Autodesk Fusion 360 part; units mm, degrees
(part 4 of 7)
  spline S889 degree 3 poles (-27.7984, 38.7746) (-27.7984, 38.6069) (-27.5964, 38.6069) (-27.5964, 38.7412) knots 0 0 0 0 1 1 1 1
  spline S890 degree 3 poles (-27.5964, 38.7412) (-27.5964, 38.8756) (-27.4117, 39.3291) (-27.4117, 38.7918) knots 0 0 0 0 1 1 1 1
  spline S891 degree 3 poles (-27.4117, 38.7918) (-27.4117, 38.6069) (-27.2945, 38.7079) (-27.2945, 38.809) knots 0 0 0 0 1 1 1 1
  line L641 (-27.2945, 38.809) -> (-27.2903, 38.9208)
  spline S892 degree 3 poles (-27.2903, 38.9208) (-27.2569, 39.1227) (-27.3826, 39.1603) (-27.4986, 39.2635) knots 0 0 0 0 1 1 1 1
  spline S893 degree 3 poles (-25.8872, 39.0304) (-25.9226, 39.5849) (-26.1773, 40.0898) (-26.6436, 40.5347) knots 0 0 0 0 1 1 1 1
  spline S894 degree 2 poles (-26.6436, 40.5347) (-26.578, 40.3295) (-26.5694, 40.0962) knots 0 0 0 1 1 1
  spline S895 degree 2 poles (-26.5694, 40.0962) (-26.6361, 40.2618) (-26.8208, 40.1779) knots 0 0 0 1 1 1
  spline S896 degree 2 poles (-26.8208, 40.1779) (-26.7198, 39.9598) (-26.7541, 39.7245) knots 0 0 0 1 1 1
  spline S897 degree 2 poles (-26.7541, 39.7245) (-26.8208, 39.8589) (-26.9218, 39.8922) knots 0 0 0 1 1 1
  spline S898 degree 2 poles (-26.9218, 39.8922) (-26.838, 39.7407) (-26.8551, 39.5063) knots 0 0 0 1 1 1
  spline S899 degree 2 poles (-26.8551, 39.5063) (-26.939, 39.6406) (-27.0905, 39.5902) knots 0 0 0 1 1 1
  spline S900 degree 2 poles (-27.0905, 39.5902) (-27.0572, 39.4731) (-27.0733, 39.271) knots 0 0 0 1 1 1
  spline S901 degree 2 poles (-27.0733, 39.271) (-27.157, 39.4407) (-27.2913, 39.3377) knots 0 0 0 1 1 1
  spline S902 degree 2 poles (-27.2913, 39.3377) (-27.0733, 39.0861) (-27.1065, 38.5651) knots 0 0 0 1 1 1
  spline S903 degree 3 poles (-27.1065, 38.5651) (-27.0077, 38.6527) (-26.9424, 38.7719) (-26.9218, 38.9025) knots 0 0 0 0 1 1 1 1
  spline S904 degree 2 poles (-26.9218, 38.9025) (-26.8884, 38.8165) (-26.8208, 38.6993) knots 0 0 0 1 1 1
  spline S905 degree 2 poles (-26.8208, 38.6993) (-26.7875, 38.768) (-26.7369, 38.9507) knots 0 0 0 1 1 1
  spline S906 degree 2 poles (-26.7369, 38.9507) (-26.6532, 38.6672) (-26.6704, 38.464) knots 0 0 0 1 1 1
  spline S907 degree 2 poles (-26.6704, 38.464) (-26.519, 38.7832) (-26.5694, 39.2366) knots 0 0 0 1 1 1
  spline S908 degree 2 poles (-26.5694, 39.2366) (-26.4018, 38.9368) (-26.4523, 38.4995) knots 0 0 0 1 1 1
  spline S909 degree 2 poles (-26.4523, 38.4995) (-26.2676, 38.8165) (-26.3675, 39.07) knots 0 0 0 1 1 1
  spline S910 degree 2 poles (-26.3675, 39.07) (-26.2343, 38.7821) (-26.2343, 38.6982) knots 0 0 0 1 1 1
  spline S911 degree 2 poles (-26.2343, 38.6982) (-26.1504, 38.9014) (-26.1, 39.1517) knots 0 0 0 1 1 1
  spline S912 degree 2 poles (-26.1, 39.1517) (-25.9323, 38.4297) (-26.1665, 37.7773) knots 0 0 0 1 1 1
  line L642 (-26.1665, 37.7773) -> (-26.1172, 37.8279)
  spline S913 degree 3 poles (-26.1172, 37.8279) (-25.9688, 38.1739) (-25.8583, 38.5897) (-25.8872, 39.0304) knots 0 0 0 0 1 1 1 1
  spline S914 degree 2 poles (-27.2569, 39.9437) (-27.3751, 40.2318) (-27.359, 40.3971) knots 0 0 0 1 1 1
  spline S915 degree 3 poles (-27.359, 40.3971) (-27.3579, 40.3961) (-27.5933, 40.1779) (-27.2569, 39.9437) knots 0 0 0 0 1 1 1 1
  spline S916 degree 2 poles (-27.1904, 40.3124) (-27.2569, 40.4134) (-27.1904, 40.5154) knots 0 0 0 1 1 1
  spline S917 degree 2 poles (-27.1904, 40.5154) (-27.1226, 40.6153) (-27.1904, 40.3124) knots 0 0 0 1 1 1
  spline S918 degree 2 poles (-25.7637, 36.4513) (-25.8141, 36.6533) (-25.7969, 36.7704) knots 0 0 0 1 1 1
  spline S919 degree 2 poles (-25.7969, 36.7704) (-25.999, 36.621) (-25.7637, 36.4513) knots 0 0 0 1 1 1
  spline S920 degree 3 poles (-25.4112, 36.7865) (-25.4264, 36.6813) (-25.3511, 36.4803) (-25.3489, 36.3965) knots 0 0 0 0 1 1 1 1
  spline S921 degree 3 poles (-25.3489, 36.3965) (-25.3877, 36.3395) (-25.4167, 36.3568) (-25.4339, 36.3815) knots 0 0 0 0 1 1 1 1
  spline S922 degree 3 poles (-25.4339, 36.3815) (-25.4565, 36.418) (-25.4687, 36.4598) (-25.4693, 36.5028) knots 0 0 0 0 1 1 1 1
  spline S923 degree 3 poles (-25.4693, 36.5028) (-25.4746, 36.621) (-25.392, 36.7618) (-25.4112, 36.7865) knots 0 0 0 0 1 1 1 1
  spline S924 degree 3 poles (-25.0246, 36.8017) (-25.0374, 36.7114) (-24.9386, 36.5083) (-24.9344, 36.3395) knots 0 0 0 0 1 1 1 1
  spline S925 degree 3 poles (-24.9344, 36.3395) (-24.9654, 36.1966) (-24.9998, 36.1944) (-25.0127, 36.2203) knots 0 0 0 0 1 1 1 1
  spline S926 degree 3 poles (-25.0127, 36.2203) (-25.0451, 36.2718) (-25.0626, 36.3313) (-25.0632, 36.3922) knots 0 0 0 0 1 1 1 1
  spline S927 degree 3 poles (-25.0632, 36.3922) (-25.0665, 36.5329) (-24.9881, 36.7489) (-25.0246, 36.8017) knots 0 0 0 0 1 1 1 1
  spline S928 degree 3 poles (-24.6389, 36.8156) (-24.6497, 36.7361) (-24.526, 36.534) (-24.5218, 36.2826) knots 0 0 0 0 1 1 1 1
  spline S929 degree 3 poles (-24.5218, 36.2826) (-24.5454, 36.0537) (-24.583, 36.0354) (-24.5927, 36.0537) knots 0 0 0 0 1 1 1 1
  spline S930 degree 3 poles (-24.5927, 36.0537) (-24.6024, 36.072) (-24.6583, 36.1547) (-24.6583, 36.2761) knots 0 0 0 0 1 1 1 1
  spline S931 degree 3 poles (-24.6583, 36.2761) (-24.6603, 36.4449) (-24.583, 36.7361) (-24.6389, 36.8156) knots 0 0 0 0 1 1 1 1
  spline S932 degree 3 poles (-24.2532, 36.8305) (-24.2618, 36.7651) (-24.1146, 36.5642) (-24.1071, 36.2278) knots 0 0 0 0 1 1 1 1
  spline S933 degree 3 poles (-24.1071, 36.2278) (-24.1243, 35.9086) (-24.163, 35.8752) (-24.1738, 35.8926) knots 0 0 0 0 1 1 1 1
  spline S934 degree 3 poles (-24.1738, 35.8926) (-24.1823, 35.9075) (-24.2521, 36.0075) (-24.2532, 36.1655) knots 0 0 0 0 1 1 1 1
  spline S935 degree 3 poles (-24.2532, 36.1655) (-24.2543, 36.3568) (-24.178, 36.7253) (-24.2532, 36.8305) knots 0 0 0 0 1 1 1 1
  spline S936 degree 3 poles (-23.8664, 36.8457) (-23.8739, 36.7951) (-23.702, 36.5921) (-23.6934, 36.1741) knots 0 0 0 0 1 1 1 1
  spline S937 degree 3 poles (-23.6934, 36.1741) (-23.7031, 35.7667) (-23.744, 35.7141) (-23.7526, 35.7292) knots 0 0 0 0 1 1 1 1
  spline S938 degree 3 poles (-23.7526, 35.7292) (-23.759, 35.7398) (-23.846, 35.8635) (-23.846, 36.0504) knots 0 0 0 0 1 1 1 1
  spline S939 degree 3 poles (-23.846, 36.0504) (-23.8471, 36.2664) (-23.7729, 36.7156) (-23.8664, 36.8457) knots 0 0 0 0 1 1 1 1
  spline S940 degree 3 poles (-23.4808, 36.8596) (-23.4862, 36.8199) (-23.2906, 36.6201) (-23.2789, 36.1149) knots 0 0 0 0 1 1 1 1
  spline S941 degree 3 poles (-23.2789, 36.1149) (-23.2831, 35.6216) (-23.3251, 35.5551) (-23.3315, 35.5648) knots 0 0 0 0 1 1 1 1
  spline S942 degree 3 poles (-23.3315, 35.5648) (-23.3368, 35.5734) (-23.44, 35.7163) (-23.44, 35.9366) knots 0 0 0 0 1 1 1 1
  spline S943 degree 3 poles (-23.44, 35.9366) (-23.4411, 36.1783) (-23.3669, 36.7048) (-23.4808, 36.8596) knots 0 0 0 0 1 1 1 1
  spline S944 degree 3 poles (-23.094, 36.8747) (-23.0984, 36.8499) (-22.8791, 36.648) (-22.8652, 36.0601) knots 0 0 0 0 1 1 1 1
  spline S945 degree 3 poles (-22.8652, 36.0601) (-22.8619, 35.4788) (-22.9071, 35.3949) (-22.9125, 35.4035) knots 0 0 0 0 1 1 1 1
  spline S946 degree 3 poles (-22.9125, 35.4035) (-22.9146, 35.4079) (-23.0339, 35.569) (-23.0339, 35.8237) knots 0 0 0 0 1 1 1 1
  spline S947 degree 3 poles (-23.0339, 35.8237) (-23.035, 36.0924) (-22.963, 36.692) (-23.094, 36.8747) knots 0 0 0 0 1 1 1 1
  spline S948 degree 3 poles (-22.7083, 36.8919) (-22.7105, 36.8768) (-22.4645, 36.6758) (-22.4505, 36.0042) knots 0 0 0 0 1 1 1 1
  spline S949 degree 3 poles (-22.4505, 36.0042) (-22.4408, 35.337) (-22.4892, 35.236) (-22.4914, 35.2381) knots 0 0 0 0 1 1 1 1
  spline S950 degree 3 poles (-22.4914, 35.2381) (-22.4925, 35.2424) (-22.6277, 35.4229) (-22.6277, 35.7099) knots 0 0 0 0 1 1 1 1
  spline S951 degree 3 poles (-22.6277, 35.7099) (-22.6277, 36.0042) (-22.5579, 36.6813) (-22.7083, 36.8919) knots 0 0 0 0 1 1 1 1
  spline S952 degree 2 poles (-22.0703, 35.0737) (-22.2217, 35.2767) (-22.2217, 35.5937) knots 0 0 0 1 1 1
  spline S953 degree 3 poles (-22.2217, 35.5937) (-22.2217, 35.9129) (-22.1551, 36.6683) (-22.3226, 36.9036) knots 0 0 0 0 1 1 1 1
  spline S954 degree 2 poles (-22.3226, 36.9036) (-22.054, 36.7038) (-22.0368, 35.9483) knots 0 0 0 1 1 1
  spline S955 degree 2 poles (-22.0368, 35.9483) (-22.0197, 35.1919) (-22.0703, 35.0737) knots 0 0 0 1 1 1
  spline S956 degree 2 poles (-21.6298, 35.1081) (-21.7812, 35.3101) (-21.7812, 35.6302) knots 0 0 0 1 1 1
  spline S957 degree 3 poles (-21.7812, 35.6302) (-21.7812, 35.9494) (-21.836, 36.6855) (-21.8812, 36.9381) knots 0 0 0 0 1 1 1 1
  spline S958 degree 2 poles (-21.8812, 36.9381) (-21.6137, 36.7361) (-21.5965, 35.9806) knots 0 0 0 1 1 1
  spline S959 degree 2 poles (-21.5965, 35.9806) (-21.5793, 35.2274) (-21.6298, 35.1081) knots 0 0 0 1 1 1
  spline S960 degree 2 poles (-21.1613, 34.805) (-21.3, 34.992) (-21.3, 35.2875) knots 0 0 0 1 1 1
  spline S961 degree 3 poles (-21.3, 35.2875) (-21.3, 35.5831) (-21.3493, 36.2697) (-21.3913, 36.5008) knots 0 0 0 0 1 1 1 1
  spline S962 degree 2 poles (-21.3913, 36.5008) (-21.1463, 36.3137) (-21.1313, 35.6152) knots 0 0 0 1 1 1
  spline S963 degree 2 poles (-21.1313, 35.6152) (-21.1162, 34.9168) (-21.1613, 34.805) knots 0 0 0 1 1 1
  spline S964 degree 3 poles (-25.2888, 34.0775) (-24.9809, 33.1248) (-24.8236, 32.13) (-24.8226, 31.1288) knots 0 0 0 0 1 1 1 1
  spline S965 degree 3 poles (-24.8226, 31.1288) (-24.8226, 28.3607) (-25.0665, 26.7047) (-25.5693, 26.0643) knots 0 0 0 0 1 1 1 1
  spline S966 degree 3 poles (-25.5693, 26.0643) (-25.6465, 25.9654) (-25.6971, 25.9718) (-25.7154, 25.9751) knots 0 0 0 0 1 1 1 1
  spline S967 degree 3 poles (-25.7154, 25.9751) (-25.8088, 25.988) (-25.9195, 26.1234) (-26.0054, 26.2706) knots 0 0 0 0 1 1 1 1
  spline S968 degree 3 poles (-26.0054, 26.2706) (-25.9607, 26.2769) (-25.9176, 26.2907) (-25.8775, 26.3114) knots 0 0 0 0 1 1 1 1
  spline S969 degree 3 poles (-25.8775, 26.3114) (-25.2888, 26.6026) (-24.9912, 28.236) (-24.9912, 31.1621) knots 0 0 0 0 1 1 1 1
  spline S970 degree 3 poles (-24.9912, 31.1621) (-24.9912, 32.3582) (-25.1169, 33.3198) (-25.2888, 34.0775) knots 0 0 0 0 1 1 1 1
  spline S971 degree 3 poles (-35.9406, 27.6708) (-35.8751, 27.5816) (-35.6215, 27.4816) (-35.8042, 27.732) knots 0 0 0 0 1 1 1 1
  spline S972 degree 3 poles (-35.8042, 27.732) (-35.8502, 27.7109) (-35.8971, 27.6919) (-35.9449, 27.6751) knots 0 0 0 0 1 1 1 1
  line L643 (-35.9449, 27.6751) -> (-35.9406, 27.6708)
  spline S973 degree 3 poles (-35.4378, 27.7041) (-35.5614, 27.7707) (-35.6054, 27.6923) (-35.5162, 27.6256) knots 0 0 0 0 1 1 1 1
  spline S974 degree 3 poles (-35.5162, 27.6256) (-35.4388, 27.5614) (-35.3522, 27.5089) (-35.2595, 27.4698) knots 0 0 0 0 1 1 1 1
  line L644 (-35.2595, 27.4698) -> (-35.2509, 27.4655)
  spline S975 degree 3 poles (-35.2509, 27.4655) (-35.2896, 27.5493) (-35.3282, 27.645) (-35.4378, 27.7041) knots 0 0 0 0 1 1 1 1
  spline S976 degree 3 poles (-33.7479, 28.9247) (-33.7587, 28.8012) (-33.8263, 28.9355) (-33.8596, 28.9806) knots 0 0 0 0 1 1 1 1
  spline S977 degree 3 poles (-33.8596, 28.9806) (-33.8929, 29.0247) (-33.9381, 28.9688) (-33.9381, 28.8796) knots 0 0 0 0 1 1 1 1
  spline S978 degree 3 poles (-33.9381, 28.8796) (-33.9381, 28.7904) (-34.0272, 28.8012) (-34.0949, 28.8571) knots 0 0 0 0 1 1 1 1
  spline S979 degree 3 poles (-34.0949, 28.8571) (-34.1615, 28.9129) (-34.2518, 28.8796) (-34.1841, 28.7668) knots 0 0 0 0 1 1 1 1
  spline S980 degree 3 poles (-34.1841, 28.7668) (-34.1175, 28.655) (-34.2174, 28.5325) (-34.3517, 28.6668) knots 0 0 0 0 1 1 1 1
  spline S981 degree 3 poles (-34.3517, 28.6668) (-34.487, 28.8012) (-34.4419, 28.6443) (-34.5085, 28.655) knots 0 0 0 0 1 1 1 1
  spline S982 degree 3 poles (-34.5085, 28.655) (-34.5762, 28.6668) (-34.6879, 28.6217) (-34.6546, 28.5551) knots 0 0 0 0 1 1 1 1
  spline S983 degree 3 poles (-34.6546, 28.5551) (-34.6213, 28.4874) (-34.487, 28.41) (-34.3968, 28.4208) knots 0 0 0 0 1 1 1 1
  spline S984 degree 3 poles (-34.3968, 28.4208) (-34.3076, 28.4315) (-34.1948, 28.2864) (-34.0605, 27.9727) knots 0 0 0 0 1 1 1 1
  spline S985 degree 3 poles (-34.0605, 27.9727) (-33.9262, 27.6589) (-34.0723, 27.8276) (-34.1615, 27.9275) knots 0 0 0 0 1 1 1 1
  spline S986 degree 3 poles (-34.1615, 27.9275) (-34.2518, 28.0285) (-34.4086, 28.0619) (-34.6095, 27.9727) knots 0 0 0 0 1 1 1 1
  spline S987 degree 3 poles (-34.6095, 27.9727) (-34.8115, 27.8835) (-34.9447, 27.8383) (-34.9232, 27.7266) knots 0 0 0 0 1 1 1 1
  spline S988 degree 3 poles (-34.9232, 27.7266) (-34.9006, 27.6148) (-34.833, 27.5579) (-34.7663, 27.4697) knots 0 0 0 0 1 1 1 1
  spline S989 degree 3 poles (-34.7663, 27.4697) (-34.6987, 27.3795) (-34.7556, 27.3129) (-34.8781, 27.4246) knots 0 0 0 0 1 1 1 1
  spline S990 degree 3 poles (-34.8781, 27.4246) (-35.0006, 27.5364) (-35.0349, 27.6374) (-35.1134, 27.6481) knots 0 0 0 0 1 1 1 1
  spline S991 degree 3 poles (-35.1134, 27.6481) (-35.1918, 27.6589) (-35.1918, 27.6041) (-35.1252, 27.5364) knots 0 0 0 0 1 1 1 1
  spline S992 degree 3 poles (-35.1252, 27.5364) (-35.0586, 27.4697) (-34.9114, 27.3687) (-35.0006, 27.3687) knots 0 0 0 0 1 1 1 1
  spline S993 degree 3 poles (-35.0006, 27.3687) (-35.0596, 27.3687) (-35.1219, 27.3591) (-35.1714, 27.3773) knots 0 0 0 0 1 1 1 1
  spline S994 degree 3 poles (-35.1714, 27.3773) (-35.1617, 27.3429) (-35.1703, 27.3118) (-35.2025, 27.301) knots 0 0 0 0 1 1 1 1
  spline S995 degree 3 poles (-35.2025, 27.301) (-35.2691, 27.2785) (-35.3142, 27.3129) (-35.3701, 27.3344) knots 0 0 0 0 1 1 1 1
  spline S996 degree 3 poles (-35.3701, 27.3344) (-35.427, 27.3569) (-35.4485, 27.2344) (-35.5613, 27.2559) knots 0 0 0 0 1 1 1 1
  spline S997 degree 3 poles (-35.5613, 27.2559) (-35.672, 27.2785) (-35.874, 27.4235) (-35.9406, 27.4912) knots 0 0 0 0 1 1 1 1
  spline S998 degree 3 poles (-35.9406, 27.4912) (-35.9868, 27.5364) (-36.063, 27.5815) (-36.0974, 27.6213) knots 0 0 0 0 1 1 1 1
  spline S999 degree 3 poles (-36.0974, 27.6213) (-36.1047, 27.6182) (-36.1118, 27.615) (-36.1189, 27.6116) knots 0 0 0 0 1 1 1 1
  spline S1000 degree 3 poles (-36.1189, 27.6116) (-36.0405, 27.5117) (-35.9094, 27.3569) (-36.0211, 27.3344) knots 0 0 0 0 1 1 1 1
  spline S1001 degree 3 poles (-36.0211, 27.3344) (-36.1329, 27.3129) (-36.1769, 27.4235) (-36.2446, 27.5031) knots 0 0 0 0 1 1 1 1
  spline S1002 degree 3 poles (-36.2446, 27.5031) (-36.2578, 27.5181) (-36.2722, 27.5321) (-36.2876, 27.545) knots 0 0 0 0 1 1 1 1
  line L645 (-36.2876, 27.545) -> (-36.5443, 27.445)
  line L646 (-36.5443, 27.445) -> (-36.2016, 27.0754)
  spline S1003 degree 3 poles (-36.2016, 27.0754) (-36.1597, 27.1184) (-36.0834, 27.1313) (-35.9653, 26.9873) knots 0 0 0 0 1 1 1 1
  spline S1004 degree 2 poles (-35.9653, 26.9873) (-35.7923, 27.1194) (-35.6398, 26.9475) knots 0 0 0 1 1 1
  line L647 (-35.6398, 26.9475) -> (-35.6269, 26.9486)
  line L648 (-35.6269, 26.9486) -> (-35.5753, 26.9529)
  spline S1005 degree 3 poles (-35.5753, 26.9529) (-35.5001, 27.0045) (-35.3518, 27.0904) (-35.3067, 26.9819) knots 0 0 0 0 1 1 1 1
  line L649 (-35.3067, 26.9819) -> (-35.296, 26.984)
  spline S1006 degree 3 poles (-35.296, 26.984) (-35.2541, 27.0227) (-35.0478, 27.2022) (-34.9576, 27.0453) knots 0 0 0 0 1 1 1 1
  spline S1007 degree 3 poles (-34.9576, 27.0453) (-34.1261, 27.2312) (-33.5492, 27.6438) (-33.2043, 28.2972) knots 0 0 0 0 1 1 1 1
  spline S1008 degree 3 poles (-33.2043, 28.2972) (-33.0088, 28.6604) (-33.0152, 28.8323) (-33.055, 28.9119) knots 0 0 0 0 1 1 1 1
  spline S1009 degree 3 poles (-33.055, 28.9119) (-33.0703, 28.9401) (-33.092, 28.9644) (-33.1184, 28.9828) knots 0 0 0 0 1 1 1 1
  line L650 (-33.1184, 28.9828) -> (-33.3408, 29.0623)
  line L651 (-33.3408, 29.0623) -> (-33.3547, 29.0645)
  spline S1010 degree 3 poles (-33.3547, 29.0645) (-33.3685, 29.0669) (-33.3816, 29.072) (-33.3934, 29.0795) knots 0 0 0 0 1 1 1 1
  spline S1011 degree 3 poles (-33.3934, 29.0795) (-33.4278, 29.0774) (-33.7372, 29.0397) (-33.7479, 28.9247) knots 0 0 0 0 1 1 1 1
  spline S1012 degree 2 poles (-36.9816, 32.1271) (-37.0826, 32.8406) (-37.4296, 33.177) knots 0 0 0 1 1 1
  spline S1013 degree 2 poles (-37.4296, 33.177) (-37.161, 32.3292) (-36.9816, 32.1271) knots 0 0 0 1 1 1
  spline S1014 degree 2 poles (-37.1664, 31.9326) (-37.4973, 33.1899) (-37.8443, 33.5252) knots 0 0 0 1 1 1
  spline S1015 degree 2 poles (-37.8443, 33.5252) (-37.3458, 32.1336) (-37.1664, 31.9326) knots 0 0 0 1 1 1
  spline S1016 degree 2 poles (-37.3823, 31.8037) (-37.5864, 32.8298) (-37.9334, 33.1684) knots 0 0 0 1 1 1
  spline S1017 degree 2 poles (-37.9334, 33.1684) (-37.5617, 32.0078) (-37.3823, 31.8037) knots 0 0 0 1 1 1
  spline S1018 degree 2 poles (-37.4177, 35.3929) (-37.4295, 35.5518) (-37.508, 35.5948) knots 0 0 0 1 1 1
  spline S1019 degree 3 poles (-37.508, 35.5948) (-37.5864, 35.641) (-37.4747, 35.4519) (-37.4177, 35.3929) knots 0 0 0 0 1 1 1 1
  spline S1020 degree 2 poles (-36.4895, 34.9016) (-36.6797, 35.1037) (-36.6689, 35.2477) knots 0 0 0 1 1 1
  spline S1021 degree 2 poles (-36.6689, 35.2477) (-36.6571, 35.3927) (-36.7463, 35.3927) knots 0 0 0 1 1 1
  spline S1022 degree 2 poles (-36.7463, 35.3927) (-36.6185, 35.4895) (-36.5121, 35.2036) knots 0 0 0 1 1 1
  spline S1023 degree 2 poles (-36.5121, 35.2036) (-36.4777, 35.1134) (-36.4895, 34.9016) knots 0 0 0 1 1 1
  line L652 (-36.612, 32.8202) -> (-36.713, 33.0222)
  spline S1024 degree 3 poles (-36.713, 33.0222) (-36.713, 33.0211) (-36.6023, 33.0544) (-36.612, 32.8202) knots 0 0 0 0 1 1 1 1
  spline S1025 degree 2 poles (-37.3683, 30.6399) (-37.5714, 31.6661) (-37.9184, 32.0014) knots 0 0 0 1 1 1
  spline S1026 degree 2 poles (-37.9184, 32.0014) (-37.5478, 30.8419) (-37.3683, 30.6399) knots 0 0 0 1 1 1
  spline S1027 degree 2 poles (-37.7078, 30.7409) (-37.7948, 31.2115) (-37.9452, 31.3641) knots 0 0 0 1 1 1
  spline S1028 degree 2 poles (-37.9452, 31.3641) (-37.7841, 30.8344) (-37.7078, 30.7409) knots 0 0 0 1 1 1
  spline S1029 degree 2 poles (-31.3082, 30.0875) (-31.2576, 29.9822) (-31.2136, 30.0155) knots 0 0 0 1 1 1
  spline S1030 degree 3 poles (-31.2136, 30.0155) (-31.1685, 30.0488) (-31.146, 30.0993) (-31.1792, 30.1498) knots 0 0 0 0 1 1 1 1
  spline S1031 degree 3 poles (-31.1792, 30.1498) (-31.2136, 30.2004) (-31.2523, 30.2057) (-31.2803, 30.1832) knots 0 0 0 0 1 1 1 1
  spline S1032 degree 3 poles (-31.2803, 30.1832) (-31.3082, 30.1617) (-31.3201, 30.1176) (-31.3082, 30.0875) knots 0 0 0 0 1 1 1 1
  spline S1033 degree 3 poles (-31.3919, 29.6846) (-31.3586, 29.6577) (-31.3479, 29.6803) (-31.3254, 29.691) knots 0 0 0 0 1 1 1 1
  spline S1034 degree 3 poles (-31.3254, 29.691) (-31.3027, 29.7017) (-31.2867, 29.7254) (-31.2974, 29.7587) knots 0 0 0 0 1 1 1 1
  spline S1035 degree 3 poles (-31.2974, 29.7587) (-31.3093, 29.792) (-31.349, 29.8479) (-31.3747, 29.8307) knots 0 0 0 0 1 1 1 1
  spline S1036 degree 3 poles (-31.3747, 29.8307) (-31.4038, 29.8146) (-31.4381, 29.7802) (-31.4253, 29.7523) knots 0 0 0 0 1 1 1 1
  spline S1037 degree 2 poles (-31.4253, 29.7523) (-31.4145, 29.7254) (-31.3919, 29.6846) knots 0 0 0 1 1 1
  spline S1038 degree 3 poles (-31.1513, 30.4185) (-31.1438, 30.3916) (-31.0944, 30.3626) (-31.061, 30.3734) knots 0 0 0 0 1 1 1 1
  spline S1039 degree 3 poles (-31.061, 30.3734) (-31.0289, 30.3852) (-30.9333, 30.4131) (-30.945, 30.4411) knots 0 0 0 0 1 1 1 1
  spline S1040 degree 3 poles (-30.945, 30.4411) (-30.9695, 30.4853) (-31.0015, 30.5249) (-31.0396, 30.5582) knots 0 0 0 0 1 1 1 1
  spline S1041 degree 3 poles (-31.0396, 30.5582) (-31.0665, 30.5818) (-31.146, 30.5582) (-31.1556, 30.541) knots 0 0 0 0 1 1 1 1
  spline S1042 degree 3 poles (-31.1556, 30.541) (-31.1685, 30.5249) (-31.1556, 30.4411) (-31.1513, 30.4185) knots 0 0 0 0 1 1 1 1
  spline S1043 degree 2 poles (-30.7829, 30.5657) (-30.7431, 30.4819) (-30.7033, 30.4916) knots 0 0 0 1 1 1
  spline S1044 degree 3 poles (-30.7033, 30.4916) (-30.6658, 30.5034) (-30.6368, 30.5206) (-30.6368, 30.5593) knots 0 0 0 0 1 1 1 1
  spline S1045 degree 3 poles (-30.6368, 30.5593) (-30.6368, 30.599) (-30.6647, 30.6323) (-30.6872, 30.6485) knots 0 0 0 0 1 1 1 1
  spline S1046 degree 3 poles (-30.6872, 30.6485) (-30.7098, 30.6657) (-30.8215, 30.598) (-30.7829, 30.5657) knots 0 0 0 0 1 1 1 1
  spline S1047 degree 3 poles (-30.6185, 30.873) (-30.5991, 30.8526) (-30.5357, 30.9053) (-30.497, 30.944) knots 0 0 0 0 1 1 1 1
  spline S1048 degree 3 poles (-30.497, 30.944) (-30.4573, 30.9848) (-30.4798, 31.0009) (-30.5143, 31.0278) knots 0 0 0 0 1 1 1 1
  spline S1049 degree 3 poles (-30.5143, 31.0278) (-30.5476, 31.0568) (-30.5584, 31.045) (-30.5862, 31.0235) knots 0 0 0 0 1 1 1 1
  spline S1050 degree 3 poles (-30.5862, 31.0235) (-30.6141, 31.0009) (-30.6689, 30.9848) (-30.6528, 30.944) knots 0 0 0 0 1 1 1 1
  spline S1051 degree 3 poles (-30.6528, 30.944) (-30.6368, 30.9053) (-30.6368, 30.8892) (-30.6185, 30.873) knots 0 0 0 0 1 1 1 1
  spline S1052 degree 3 poles (-30.4305, 30.6248) (-30.4078, 30.6087) (-30.3972, 30.5861) (-30.3638, 30.6087) knots 0 0 0 0 1 1 1 1
  spline S1053 degree 3 poles (-30.3638, 30.6087) (-30.3306, 30.6313) (-30.3004, 30.6753) (-30.3081, 30.7097) knots 0 0 0 0 1 1 1 1
  spline S1054 degree 3 poles (-30.3081, 30.7097) (-30.3134, 30.7419) (-30.3349, 30.7419) (-30.3638, 30.7419) knots 0 0 0 0 1 1 1 1
  spline S1055 degree 3 poles (-30.3638, 30.7419) (-30.3907, 30.7419) (-30.4853, 30.6657) (-30.4477, 30.6302) knots 0 0 0 0 1 1 1 1
  line L653 (-30.4477, 30.6302) -> (-30.4305, 30.6248)
  spline S1056 degree 3 poles (-30.2564, 31.0622) (-30.2242, 31.0235) (-30.1791, 31.0235) (-30.1899, 31.0848) knots 0 0 0 0 1 1 1 1
  spline S1057 degree 3 poles (-30.1899, 31.0848) (-30.2016, 31.146) (-30.2242, 31.1524) (-30.2403, 31.1578) knots 0 0 0 0 1 1 1 1
  spline S1058 degree 3 poles (-30.2403, 31.1578) (-30.2564, 31.1621) (-30.2898, 31.103) (-30.2564, 31.0622) knots 0 0 0 0 1 1 1 1
  spline S1059 degree 3 poles (-30.2458, 30.4131) (-30.2242, 30.3884) (-30.2124, 30.3401) (-30.1727, 30.368) knots 0 0 0 0 1 1 1 1
  spline S1060 degree 3 poles (-30.1727, 30.368) (-30.1329, 30.397) (-30.0835, 30.4303) (-30.1115, 30.4518) knots 0 0 0 0 1 1 1 1
  spline S1061 degree 3 poles (-30.1115, 30.4518) (-30.1393, 30.4744) (-30.1393, 30.5023) (-30.1661, 30.5195) knots 0 0 0 0 1 1 1 1
  spline S1062 degree 3 poles (-30.1661, 30.5195) (-30.1952, 30.5367) (-30.279, 30.4518) (-30.2458, 30.4131) knots 0 0 0 0 1 1 1 1
  spline S1063 degree 3 poles (-31.0214, 29.8479) (-31.0042, 29.8124) (-30.9601, 29.7974) (-30.9333, 29.8361) knots 0 0 0 0 1 1 1 1
  spline S1064 degree 3 poles (-30.9333, 29.8361) (-30.9053, 29.8758) (-30.9214, 29.9145) (-30.9505, 29.9435) knots 0 0 0 0 1 1 1 1
  spline S1065 degree 3 poles (-30.9505, 29.9435) (-30.9784, 29.9704) (-31.0621, 29.9263) (-31.0214, 29.8479) knots 0 0 0 0 1 1 1 1
  spline S1066 degree 3 poles (-31.5048, 29.4116) (-31.4954, 29.4032) (-31.4842, 29.3974) (-31.4718, 29.3948) knots 0 0 0 0 1 1 1 1
  spline S1067 degree 3 poles (-31.4718, 29.3948) (-31.4597, 29.3922) (-31.4469, 29.3929) (-31.435, 29.3968) knots 0 0 0 0 1 1 1 1
  spline S1068 degree 3 poles (-31.435, 29.3968) (-31.4231, 29.4008) (-31.4124, 29.4078) (-31.4041, 29.4172) knots 0 0 0 0 1 1 1 1
  spline S1069 degree 3 poles (-31.4041, 29.4172) (-31.3958, 29.4266) (-31.3902, 29.438) (-31.3877, 29.4503) knots 0 0 0 0 1 1 1 1
  spline S1070 degree 3 poles (-31.3877, 29.4503) (-31.3747, 29.5008) (-31.4209, 29.5234) (-31.4381, 29.5406) knots 0 0 0 0 1 1 1 1
  spline S1071 degree 3 poles (-31.4381, 29.5406) (-31.4553, 29.5567) (-31.5832, 29.5567) (-31.5499, 29.5008) knots 0 0 0 0 1 1 1 1
  spline S1072 degree 2 poles (-31.5499, 29.5008) (-31.5156, 29.4449) (-31.5048, 29.4116) knots 0 0 0 1 1 1
  spline S1073 degree 3 poles (-30.0545, 32.4968) (-30.0158, 32.4613) (-29.9772, 32.428) (-29.9772, 32.4678) knots 0 0 0 0 1 1 1 1
  spline S1074 degree 3 poles (-29.9772, 32.4678) (-29.9772, 32.5054) (-29.9825, 32.5344) (-30.0276, 32.5559) knots 0 0 0 0 1 1 1 1
  spline S1075 degree 3 poles (-30.0276, 32.5559) (-30.0717, 32.5784) (-30.0888, 32.5215) (-30.0545, 32.4968) knots 0 0 0 0 1 1 1 1
  spline S1076 degree 3 poles (-29.6129, 31.4426) (-29.5807, 31.3878) (-29.5292, 31.3921) (-29.5066, 31.4308) knots 0 0 0 0 1 1 1 1
  spline S1077 degree 3 poles (-29.5066, 31.4308) (-29.4841, 31.4727) (-29.5002, 31.4867) (-29.5387, 31.5167) knots 0 0 0 0 1 1 1 1
  spline S1078 degree 3 poles (-29.5387, 31.5167) (-29.5807, 31.5436) (-29.658, 31.5232) (-29.6129, 31.4426) knots 0 0 0 0 1 1 1 1
  spline S1079 degree 3 poles (-29.8139, 33.2833) (-29.7945, 33.2393) (-29.7687, 33.206) (-29.7516, 33.2436) knots 0 0 0 0 1 1 1 1
  spline S1080 degree 3 poles (-29.7516, 33.2436) (-29.7355, 33.2833) (-29.7247, 33.3275) (-29.758, 33.3533) knots 0 0 0 0 1 1 1 1
  spline S1081 degree 3 poles (-29.758, 33.3533) (-29.7923, 33.3737) (-29.8363, 33.3339) (-29.8139, 33.2833) knots 0 0 0 0 1 1 1 1
  spline S1082 degree 3 poles (-29.6408, 33.6595) (-29.6184, 33.6218) (-29.5904, 33.5584) (-29.5796, 33.6132) knots 0 0 0 0 1 1 1 1
  spline S1083 degree 3 poles (-29.5796, 33.6132) (-29.5667, 33.6702) (-29.5334, 33.6863) (-29.5667, 33.7143) knots 0 0 0 0 1 1 1 1
  spline S1084 degree 3 poles (-29.5667, 33.7143) (-29.6021, 33.7433) (-29.6635, 33.6993) (-29.6408, 33.6595) knots 0 0 0 0 1 1 1 1
  spline S1085 degree 3 poles (-28.0347, 32.4774) (-28.0058, 32.4291) (-27.9724, 32.3829) (-27.9455, 32.4269) knots 0 0 0 0 1 1 1 1
  spline S1086 degree 3 poles (-27.9455, 32.4269) (-27.9177, 32.471) (-27.9059, 32.4602) (-27.951, 32.5215) knots 0 0 0 0 1 1 1 1
  spline S1087 degree 3 poles (-27.951, 32.5215) (-27.9961, 32.5849) (-28.067, 32.5344) (-28.0347, 32.4774) knots 0 0 0 0 1 1 1 1
  spline S1088 degree 3 poles (-29.5173, 35.0092) (-29.4947, 34.9652) (-29.4507, 34.9404) (-29.4507, 34.9738) knots 0 0 0 0 1 1 1 1
  spline S1089 degree 3 poles (-29.4507, 34.9738) (-29.4507, 35.0092) (-29.4614, 35.0372) (-29.4841, 35.0489) knots 0 0 0 0 1 1 1 1
  spline S1090 degree 3 poles (-29.4841, 35.0489) (-29.5066, 35.0575) (-29.5292, 35.0295) (-29.5173, 35.0092) knots 0 0 0 0 1 1 1 1
  spline S1091 degree 2 poles (-25.4317, 31.2126) (-25.5283, 31.3136) (-25.6069, 31.4544) knots 0 0 0 1 1 1
  spline S1092 degree 3 poles (-25.6069, 31.4544) (-25.6842, 31.5941) (-25.6455, 31.6156) (-25.5499, 31.4813) knots 0 0 0 0 1 1 1 1
  spline S1093 degree 3 poles (-25.5499, 31.4813) (-25.4554, 31.3469) (-25.3436, 31.0955) (-25.4317, 31.2126) knots 0 0 0 0 1 1 1 1
  spline S1094 degree 3 poles (-26.1934, 31.6382) (-26.3083, 31.7413) (-26.3664, 31.8252) (-26.3169, 31.8799) knots 0 0 0 0 1 1 1 1
  spline S1095 degree 3 poles (-26.3169, 31.8799) (-26.2665, 31.9348) (-26.2095, 31.9133) (-26.1709, 31.8466) knots 0 0 0 0 1 1 1 1
  spline S1096 degree 3 poles (-26.1709, 31.8466) (-26.1322, 31.78) (-26.0989, 31.5565) (-26.1934, 31.6382) knots 0 0 0 0 1 1 1 1
  spline S1097 degree 3 poles (-26.4791, 32.0035) (-26.5738, 32.0744) (-26.6704, 32.2088) (-26.6253, 32.2367) knots 0 0 0 0 1 1 1 1
  spline S1098 degree 3 poles (-26.6253, 32.2367) (-26.5802, 32.2657) (-26.5403, 32.3624) (-26.4791, 32.2432) knots 0 0 0 0 1 1 1 1
  spline S1099 degree 3 poles (-26.4791, 32.2432) (-26.4179, 32.1271) (-26.3567, 31.9068) (-26.4791, 32.0035) knots 0 0 0 0 1 1 1 1
  spline S1100 degree 3 poles (-26.7145, 32.4441) (-26.7821, 32.5215) (-26.8884, 32.5677) (-26.8434, 32.6118) knots 0 0 0 0 1 1 1 1
  spline S1101 degree 3 poles (-26.8434, 32.6118) (-26.7983, 32.6557) (-26.7821, 32.7526) (-26.7252, 32.6687) knots 0 0 0 0 1 1 1 1
  spline S1102 degree 3 poles (-26.7252, 32.6687) (-26.6704, 32.5849) (-26.6414, 32.3624) (-26.7145, 32.4441) knots 0 0 0 0 1 1 1 1
  spline S1103 degree 3 poles (-26.3567, 32.4506) (-26.4146, 32.5075) (-26.4684, 32.5408) (-26.419, 32.5849) knots 0 0 0 0 1 1 1 1
  spline S1104 degree 3 poles (-26.419, 32.5849) (-26.3675, 32.6311) (-26.3459, 32.5849) (-26.3072, 32.5344) knots 0 0 0 0 1 1 1 1
  spline S1105 degree 3 poles (-26.3072, 32.5344) (-26.2687, 32.4839) (-26.3063, 32.4) (-26.3567, 32.4506) knots 0 0 0 0 1 1 1 1
  spline S1106 degree 3 poles (-26.8261, 32.0744) (-26.8809, 32.14) (-26.9218, 32.1937) (-26.8767, 32.2217) knots 0 0 0 0 1 1 1 1
  spline S1107 degree 3 poles (-26.8767, 32.2217) (-26.8316, 32.2496) (-26.8659, 32.2872) (-26.7928, 32.1991) knots 0 0 0 0 1 1 1 1
  spline S1108 degree 3 poles (-26.7928, 32.1991) (-26.7198, 32.1088) (-26.7649, 32.0035) (-26.8261, 32.0744) knots 0 0 0 0 1 1 1 1
  spline S1109 degree 3 poles (-27.0894, 32.0347) (-27.1389, 32.1099) (-27.1732, 32.1271) (-27.1453, 32.1475) knots 0 0 0 0 1 1 1 1
  spline S1110 degree 3 poles (-27.1453, 32.1475) (-27.1173, 32.1679) (-27.0775, 32.169) (-27.0506, 32.1185) knots 0 0 0 0 1 1 1 1
  spline S1111 degree 3 poles (-27.0506, 32.1185) (-27.0229, 32.068) (-27.0775, 32.0186) (-27.0894, 32.0347) knots 0 0 0 0 1 1 1 1
  spline S1112 degree 3 poles (-26.6478, 32.8804) (-26.6984, 32.9309) (-26.7145, 32.9438) (-26.6973, 32.9643) knots 0 0 0 0 1 1 1 1
  spline S1113 degree 3 poles (-26.6973, 32.9643) (-26.6812, 32.9868) (-26.635, 32.9643) (-26.6198, 32.9427) knots 0 0 0 0 1 1 1 1
  spline S1114 degree 3 poles (-26.6198, 32.9427) (-26.6027, 32.9201) (-26.6134, 32.847) (-26.6478, 32.8804) knots 0 0 0 0 1 1 1 1
  spline S1115 degree 3 poles (-26.3213, 32.8202) (-26.3728, 32.8686) (-26.3556, 32.9256) (-26.3277, 32.932) knots 0 0 0 0 1 1 1 1
  spline S1116 degree 3 poles (-26.3277, 32.932) (-26.3008, 32.9384) (-26.2612, 32.8653) (-26.2449, 32.8245) knots 0 0 0 0 1 1 1 1
  spline S1117 degree 3 poles (-26.2449, 32.8245) (-26.2277, 32.7858) (-26.2889, 32.7858) (-26.3213, 32.8202) knots 0 0 0 0 1 1 1 1
  spline S1118 degree 3 poles (-26.5802, 33.2833) (-26.6242, 33.3189) (-26.6361, 33.3275) (-26.6081, 33.3522) knots 0 0 0 0 1 1 1 1
  spline S1119 degree 3 poles (-26.6081, 33.3522) (-26.5802, 33.3737) (-26.5469, 33.3458) (-26.5243, 33.3102) knots 0 0 0 0 1 1 1 1
  spline S1120 degree 3 poles (-26.5243, 33.3102) (-26.5007, 33.278) (-26.5522, 33.263) (-26.5802, 33.2833) knots 0 0 0 0 1 1 1 1
  spline S1121 degree 3 poles (-26.882, 33.2899) (-26.9132, 33.3253) (-26.9432, 33.3564) (-26.9164, 33.3672) knots 0 0 0 0 1 1 1 1
  spline S1122 degree 3 poles (-26.9164, 33.3672) (-26.8886, 33.3779) (-26.8712, 33.3564) (-26.8487, 33.3339) knots 0 0 0 0 1 1 1 1
  spline S1123 degree 3 poles (-26.8487, 33.3339) (-26.8261, 33.3113) (-26.8541, 33.2564) (-26.882, 33.2899) knots 0 0 0 0 1 1 1 1
  spline S1124 degree 3 poles (-25.422, 29.8253) (-25.3661, 29.7522) (-25.3157, 29.6963) (-25.3104, 29.8532) knots 0 0 0 0 1 1 1 1
  spline S1125 degree 3 poles (-25.3104, 29.8532) (-25.3049, 30.0101) (-25.3823, 30.1498) (-25.466, 30.2519) knots 0 0 0 0 1 1 1 1
  spline S1126 degree 3 poles (-25.466, 30.2519) (-25.551, 30.3529) (-25.4843, 30.4357) (-25.4447, 30.3572) knots 0 0 0 0 1 1 1 1
  spline S1127 degree 3 poles (-25.4447, 30.3572) (-25.4048, 30.2798) (-25.2932, 30.2573) (-25.3049, 30.3357) knots 0 0 0 0 1 1 1 1
  spline S1128 degree 3 poles (-25.3049, 30.3357) (-25.3157, 30.4142) (-25.3436, 30.498) (-25.4618, 30.671) knots 0 0 0 0 1 1 1 1
  spline S1129 degree 3 poles (-25.4618, 30.671) (-25.5789, 30.8451) (-25.4618, 30.8397) (-25.3952, 30.7602) knots 0 0 0 0 1 1 1 1
  spline S1130 degree 3 poles (-25.3952, 30.7602) (-25.3286, 30.6828) (-25.2877, 30.6602) (-25.306, 30.7269) knots 0 0 0 0 1 1 1 1
  spline S1131 degree 3 poles (-25.306, 30.7269) (-25.3221, 30.7946) (-25.5629, 31.1932) (-25.6692, 31.3609) knots 0 0 0 0 1 1 1 1
  spline S1132 degree 3 poles (-25.6692, 31.3609) (-25.7755, 31.5285) (-25.7421, 31.3985) (-25.7315, 31.3147) knots 0 0 0 0 1 1 1 1
  spline S1133 degree 3 poles (-25.7315, 31.3147) (-25.7207, 31.2309) (-25.7755, 31.2588) (-25.8324, 31.3147) knots 0 0 0 0 1 1 1 1
  spline S1134 degree 3 poles (-25.8324, 31.3147) (-25.8883, 31.3716) (-25.9162, 31.4232) (-26.0173, 31.5049) knots 0 0 0 0 1 1 1 1
  spline S1135 degree 3 poles (-26.0173, 31.5049) (-26.1183, 31.5887) (-26.0226, 31.2534) (-25.9785, 31.1245) knots 0 0 0 0 1 1 1 1
  spline S1136 degree 3 poles (-25.9785, 31.1245) (-25.9334, 30.9955) (-25.9721, 30.9622) (-26.0549, 31.046) knots 0 0 0 0 1 1 1 1
  spline S1137 degree 3 poles (-26.0549, 31.046) (-26.1386, 31.1298) (-26.3869, 31.6123) (-26.5093, 31.7467) knots 0 0 0 0 1 1 1 1
  spline S1138 degree 3 poles (-26.5093, 31.7467) (-26.6317, 31.881) (-26.6887, 31.7929) (-26.592, 31.6564) knots 0 0 0 0 1 1 1 1
  spline S1139 degree 3 poles (-26.592, 31.6564) (-26.4343, 31.4147) (-26.2874, 31.1662) (-26.1515, 30.9117) knots 0 0 0 0 1 1 1 1
  spline S1140 degree 3 poles (-26.1515, 30.9117) (-26.0732, 30.7602) (-26.1386, 30.656) (-26.2127, 30.7774) knots 0 0 0 0 1 1 1 1
  spline S1141 degree 3 poles (-26.2127, 30.7774) (-26.2858, 30.901) (-26.4706, 31.2255) (-26.593, 31.3652) knots 0 0 0 0 1 1 1 1
  spline S1142 degree 3 poles (-26.593, 31.3652) (-26.7166, 31.5049) (-26.7563, 31.4737) (-26.7059, 31.348) knots 0 0 0 0 1 1 1 1
  spline S1143 degree 3 poles (-26.7059, 31.348) (-26.6553, 31.2255) (-26.4985, 30.945) (-26.476, 30.7774) knots 0 0 0 0 1 1 1 1
  spline S1144 degree 3 poles (-26.476, 30.7774) (-26.4534, 30.6097) (-26.5157, 30.6495) (-26.5877, 30.7956) knots 0 0 0 0 1 1 1 1
  spline S1145 degree 3 poles (-26.5877, 30.7956) (-26.6596, 30.9418) (-27.0238, 31.5575) (-27.2021, 31.8649) knots 0 0 0 0 1 1 1 1
  spline S1146 degree 3 poles (-27.2021, 31.8649) (-27.3815, 32.1711) (-27.3762, 31.9863) (-27.3311, 31.9089) knots 0 0 0 0 1 1 1 1
  spline S1147 degree 3 poles (-27.3311, 31.9089) (-27.286, 31.8316) (-26.895, 31.0643) (-26.8391, 30.902) knots 0 0 0 0 1 1 1 1
  spline S1148 degree 3 poles (-26.8391, 30.902) (-26.7832, 30.7408) (-26.867, 30.7785) (-26.9401, 30.8752) knots 0 0 0 0 1 1 1 1
  spline S1149 degree 3 poles (-26.9401, 30.8752) (-27.0121, 30.9708) (-27.5944, 31.9992) (-27.6738, 32.0959) knots 0 0 0 0 1 1 1 1
  spline S1150 degree 3 poles (-27.6738, 32.0959) (-27.75, 32.1905) (-27.763, 32.14) (-27.7297, 32.0497) knots 0 0 0 0 1 1 1 1
  spline S1151 degree 3 poles (-27.7297, 32.0497) (-27.6963, 31.9616) (-27.2817, 31.1599) (-27.243, 31.0138) knots 0 0 0 0 1 1 1 1
  spline S1152 degree 3 poles (-27.243, 31.0138) (-27.2032, 30.8687) (-27.2871, 30.8967) (-27.3547, 30.9966) knots 0 0 0 0 1 1 1 1
  spline S1153 degree 3 poles (-27.3547, 30.9966) (-27.4224, 31.0965) (-27.9488, 31.9326) (-28.0197, 32.0368) knots 0 0 0 0 1 1 1 1
  spline S1154 degree 3 poles (-28.0197, 32.0368) (-28.0928, 32.1464) (-28.1938, 32.1034) (-28.1164, 31.982) knots 0 0 0 0 1 1 1 1
  spline S1155 degree 3 poles (-28.1164, 31.982) (-28.038, 31.8584) (-27.5008, 30.7956) (-27.4385, 30.6721) knots 0 0 0 0 1 1 1 1
  spline S1156 degree 3 poles (-27.4385, 30.6721) (-27.3773, 30.5496) (-27.4277, 30.4926) (-27.489, 30.5775) knots 0 0 0 0 1 1 1 1
  spline S1157 degree 3 poles (-27.489, 30.5775) (-27.5513, 30.6613) (-28.2678, 31.881) (-28.3614, 31.9992) knots 0 0 0 0 1 1 1 1
  spline S1158 degree 3 poles (-28.3614, 31.9992) (-28.4569, 32.1163) (-28.4849, 32.0164) (-28.4397, 31.8917) knots 0 0 0 0 1 1 1 1
  spline S1159 degree 3 poles (-28.4397, 31.8917) (-28.3957, 31.7682) (-27.9198, 30.8784) (-27.8586, 30.7838) knots 0 0 0 0 1 1 1 1
  spline S1160 degree 3 poles (-27.8586, 30.7838) (-27.7952, 30.6882) (-27.864, 30.6721) (-27.9477, 30.7398) knots 0 0 0 0 1 1 1 1
  spline S1161 degree 3 poles (-27.9477, 30.7398) (-28.0316, 30.8064) (-28.5516, 31.7295) (-28.6418, 31.8176) knots 0 0 0 0 1 1 1 1
  spline S1162 degree 3 poles (-28.6418, 31.8176) (-28.731, 31.9078) (-28.7814, 31.9014) (-28.7138, 31.7424) knots 0 0 0 0 1 1 1 1
  spline S1163 degree 3 poles (-28.7138, 31.7424) (-28.6471, 31.579) (-28.3173, 30.9515) (-28.2722, 30.8505) knots 0 0 0 0 1 1 1 1
  spline S1164 degree 3 poles (-28.2722, 30.8505) (-28.2271, 30.7494) (-28.2443, 30.6667) (-28.3109, 30.772) knots 0 0 0 0 1 1 1 1
  spline S1165 degree 3 poles (-28.3109, 30.772) (-28.3774, 30.8784) (-28.8212, 31.6231) (-28.9104, 31.7069) knots 0 0 0 0 1 1 1 1
  spline S1166 degree 3 poles (-28.9104, 31.7069) (-28.9995, 31.7929) (-29.0726, 31.7972) (-28.9995, 31.6671) knots 0 0 0 0 1 1 1 1
  spline S1167 degree 3 poles (-28.9995, 31.6671) (-28.9276, 31.5393) (-28.5912, 30.7903) (-28.5698, 30.6678) knots 0 0 0 0 1 1 1 1
  spline S1168 degree 3 poles (-28.5698, 30.6678) (-28.5472, 30.5431) (-28.5633, 30.5098) (-28.6256, 30.6269) knots 0 0 0 0 1 1 1 1
  spline S1169 degree 3 poles (-28.6256, 30.6269) (-28.6879, 30.7441) (-29.0284, 31.3448) (-29.0907, 31.406) knots 0 0 0 0 1 1 1 1
  spline S1170 degree 3 poles (-29.0907, 31.406) (-29.1532, 31.4683) (-29.2294, 31.4748) (-29.1627, 31.3791) knots 0 0 0 0 1 1 1 1
  spline S1171 degree 3 poles (-29.1627, 31.3791) (-29.0951, 31.2824) (-28.877, 30.7408) (-28.8265, 30.628) knots 0 0 0 0 1 1 1 1
  spline S1172 degree 3 poles (-28.8265, 30.628) (-28.7772, 30.5173) (-28.906, 30.4604) (-28.9447, 30.5893) knots 0 0 0 0 1 1 1 1
  spline S1173 degree 3 poles (-28.9447, 30.5893) (-28.9833, 30.7193) (-29.1349, 30.9977) (-29.2358, 31.1492) knots 0 0 0 0 1 1 1 1
  spline S1174 degree 3 poles (-29.2358, 31.1492) (-29.3379, 31.3007) (-29.4722, 31.0826) (-29.4088, 30.9923) knots 0 0 0 0 1 1 1 1
  spline S1175 degree 3 poles (-29.4088, 30.9923) (-29.3476, 30.9031) (-29.2294, 30.6065) (-29.1466, 30.4496) knots 0 0 0 0 1 1 1 1
  spline S1176 degree 3 poles (-29.1466, 30.4496) (-29.0629, 30.2927) (-29.1295, 30.2207) (-29.181, 30.2992) knots 0 0 0 0 1 1 1 1
  spline S1177 degree 3 poles (-29.181, 30.2992) (-29.2294, 30.3766) (-29.4218, 30.7516) (-29.4539, 30.8128) knots 0 0 0 0 1 1 1 1
  spline S1178 degree 3 poles (-29.4539, 30.8128) (-29.4872, 30.8762) (-29.6107, 30.7236) (-29.6279, 30.685) knots 0 0 0 0 1 1 1 1
  spline S1179 degree 3 poles (-29.6279, 30.685) (-29.6452, 30.6452) (-29.5044, 30.4271) (-29.4711, 30.3432) knots 0 0 0 0 1 1 1 1
  spline S1180 degree 3 poles (-29.4711, 30.3432) (-29.4368, 30.2594) (-29.4764, 30.1702) (-29.5205, 30.2089) knots 0 0 0 0 1 1 1 1
  spline S1181 degree 3 poles (-29.5205, 30.2089) (-29.5787, 30.2772) (-29.6277, 30.3527) (-29.6666, 30.4335) knots 0 0 0 0 1 1 1 1
  spline S1182 degree 3 poles (-29.6666, 30.4335) (-29.6946, 30.4894) (-29.7622, 30.5001) (-29.8289, 30.5227) knots 0 0 0 0 1 1 1 1
  spline S1183 degree 3 poles (-29.8289, 30.5227) (-29.8955, 30.5442) (-29.8515, 30.6903) (-29.8997, 30.7623) knots 0 0 0 0 1 1 1 1
  spline S1184 degree 3 poles (-29.8997, 30.7623) (-29.9513, 30.8365) (-29.9578, 30.858) (-30.034, 30.9257) knots 0 0 0 0 1 1 1 1
  spline S1185 degree 3 poles (-30.034, 30.9257) (-30.1135, 30.9923) (-30.1071, 30.8128) (-30.0684, 30.7688) knots 0 0 0 0 1 1 1 1
  spline S1186 degree 3 poles (-30.0684, 30.7688) (-30.0298, 30.7236) (-29.9675, 30.6011) (-29.9341, 30.5614) knots 0 0 0 0 1 1 1 1
  spline S1187 degree 3 poles (-29.9341, 30.5614) (-29.8997, 30.5227) (-29.9567, 30.4056) (-29.9847, 30.3325) knots 0 0 0 0 1 1 1 1
  spline S1188 degree 3 poles (-29.9847, 30.3325) (-30.0126, 30.2594) (-30.0803, 30.1982) (-30.1243, 30.1863) knots 0 0 0 0 1 1 1 1
  spline S1189 degree 3 poles (-30.1243, 30.1863) (-30.1683, 30.1756) (-30.2918, 30.2089) (-30.337, 30.2659) knots 0 0 0 0 1 1 1 1
  spline S1190 degree 3 poles (-30.337, 30.2659) (-30.3794, 30.3236) (-30.4327, 30.3725) (-30.4939, 30.4099) knots 0 0 0 0 1 1 1 1
  spline S1191 degree 3 poles (-30.4939, 30.4099) (-30.5443, 30.4335) (-30.5659, 30.3658) (-30.5498, 30.3099) knots 0 0 0 0 1 1 1 1
  spline S1192 degree 3 poles (-30.5498, 30.3099) (-30.5336, 30.2541) (-30.4327, 30.1649) (-30.3821, 30.1315) knots 0 0 0 0 1 1 1 1
  spline S1193 degree 3 poles (-30.3821, 30.1315) (-30.3317, 30.0972) (-30.4488, 29.9349) (-30.5047, 29.9016) knots 0 0 0 0 1 1 1 1
  spline S1194 degree 3 poles (-30.5047, 29.9016) (-30.5604, 29.8672) (-30.567, 29.9403) (-30.5776, 30.0069) knots 0 0 0 0 1 1 1 1
  spline S1195 degree 3 poles (-30.5776, 30.0069) (-30.5884, 30.0746) (-30.6841, 30.1982) (-30.7387, 30.2541) knots 0 0 0 0 1 1 1 1
  spline S1196 degree 3 poles (-30.7387, 30.2541) (-30.7946, 30.3099) (-30.8054, 30.3432) (-30.8677, 30.3099) knots 0 0 0 0 1 1 1 1
  spline S1197 degree 3 poles (-30.8677, 30.3099) (-30.9289, 30.2755) (-30.9289, 30.2089) (-30.8893, 30.153) knots 0 0 0 0 1 1 1 1
  spline S1198 degree 3 poles (-30.8893, 30.153) (-30.8266, 30.0733) (-30.7562, 30.0002) (-30.6786, 29.9349) knots 0 0 0 0 1 1 1 1
  spline S1199 degree 3 poles (-30.6786, 29.9349) (-30.6443, 29.9134) (-30.5776, 29.8565) (-30.5831, 29.8006) knots 0 0 0 0 1 1 1 1
  spline S1200 degree 3 poles (-30.5831, 29.8006) (-30.5884, 29.7447) (-30.7002, 29.7791) (-30.7442, 29.7619) knots 0 0 0 0 1 1 1 1
  spline S1201 degree 3 poles (-30.7442, 29.7619) (-30.7893, 29.7447) (-30.8279, 29.7049) (-30.8279, 29.6491) knots 0 0 0 0 1 1 1 1
  spline S1202 degree 3 poles (-30.8279, 29.6491) (-30.8279, 29.5942) (-30.8279, 29.5652) (-30.8849, 29.5599) knots 0 0 0 0 1 1 1 1
  spline S1203 degree 3 poles (-30.8849, 29.5599) (-30.9408, 29.5534) (-31.0073, 29.5437) (-31.0073, 29.5996) knots 0 0 0 0 1 1 1 1
  spline S1204 degree 3 poles (-31.0073, 29.5996) (-31.0073, 29.6544) (-31.0524, 29.6662) (-31.1244, 29.6781) knots 0 0 0 0 1 1 1 1
  spline S1205 degree 3 poles (-31.1244, 29.6781) (-31.1964, 29.6877) (-31.1964, 29.476) (-31.1964, 29.4148) knots 0 0 0 0 1 1 1 1
  spline S1206 degree 3 poles (-31.1964, 29.4148) (-31.1964, 29.3525) (-31.2404, 29.3858) (-31.3038, 29.403) knots 0 0 0 0 1 1 1 1
  spline S1207 degree 3 poles (-31.3038, 29.403) (-31.365, 29.4191) (-31.3307, 29.3353) (-31.3747, 29.3256) knots 0 0 0 0 1 1 1 1
  spline S1208 degree 3 poles (-31.3747, 29.3256) (-31.4209, 29.3138) (-31.6939, 29.2966) (-31.7401, 29.3138) knots 0 0 0 0 1 1 1 1
  spline S1209 degree 3 poles (-31.7401, 29.3138) (-31.7852, 29.331) (-31.767, 29.3697) (-31.7852, 29.4094) knots 0 0 0 0 1 1 1 1
  spline S1210 degree 3 poles (-31.7852, 29.4094) (-31.8013, 29.4481) (-31.8518, 29.476) (-31.8797, 29.4868) knots 0 0 0 0 1 1 1 1
  spline S1211 degree 3 poles (-31.8797, 29.4868) (-31.9077, 29.4986) (-31.9581, 29.4309) (-31.9625, 29.3976) knots 0 0 0 0 1 1 1 1
  spline S1212 degree 3 poles (-31.9625, 29.3976) (-31.97, 29.3643) (-31.9581, 29.3417) (-31.9356, 29.3191) knots 0 0 0 0 1 1 1 1
  spline S1213 degree 2 poles (-31.9356, 29.3191) (-31.913, 29.2966) (-31.8346, 29.2686) knots 0 0 0 1 1 1
  spline S1214 degree 3 poles (-31.8346, 29.2686) (-31.7906, 29.1966) (-31.8174, 29.1236) (-31.8625, 29.1236) knots 0 0 0 0 1 1 1 1
  spline S1215 degree 3 poles (-31.8625, 29.1236) (-31.9077, 29.1236) (-31.9291, 29.1236) (-31.9625, 29.1741) knots 0 0 0 0 1 1 1 1
  spline S1216 degree 3 poles (-31.9625, 29.1741) (-31.9968, 29.2246) (-32.0301, 29.1676) (-32.0752, 29.1504) knots 0 0 0 0 1 1 1 1
  spline S1217 degree 3 poles (-32.0752, 29.1504) (-32.1192, 29.1343) (-32.1364, 29.101) (-32.1364, 29.0226) knots 0 0 0 0 1 1 1 1
  spline S1218 degree 3 poles (-32.1364, 29.0226) (-32.1364, 28.9441) (-32.231, 28.9388) (-32.2934, 28.8603) knots 0 0 0 0 1 1 1 1
  spline S1219 degree 3 poles (-32.2934, 28.8603) (-32.3546, 28.7819) (-32.3546, 28.9162) (-32.3546, 29.0451) knots 0 0 0 0 1 1 1 1
  spline S1220 degree 3 poles (-32.3546, 29.0451) (-32.3546, 29.1741) (-32.462, 29.0849) (-32.5565, 29.0118) knots 0 0 0 0 1 1 1 1
  spline S1221 degree 3 poles (-32.5565, 29.0118) (-32.6461, 28.9399) (-32.7271, 28.8581) (-32.7982, 28.7679) knots 0 0 0 0 1 1 1 1
  spline S1222 degree 3 poles (-32.7982, 28.7679) (-32.8068, 28.611) (-32.8713, 28.4219) (-32.9948, 28.1897) knots 0 0 0 0 1 1 1 1
  line L654 (-32.9948, 28.1897) -> (-33.0013, 28.1812)
  spline S1223 degree 3 poles (-33.0013, 28.1812) (-32.9421, 27.7943) (-32.2782, 26.9314) (-32.1344, 26.753) knots 0 0 0 0 1 1 1 1
  line L655 (-32.1344, 26.753) -> (-32.001, 26.753)
  spline S1224 degree 3 poles (-32.001, 26.753) (-32.1225, 26.9798) (-32.4845, 27.6406) (-32.5221, 27.7685) knots 0 0 0 0 1 1 1 1
  spline S1225 degree 3 poles (-32.5221, 27.7685) (-32.5672, 27.92) (-32.4942, 28.0039) (-32.449, 27.8308) knots 0 0 0 0 1 1 1 1
  spline S1226 degree 3 poles (-32.449, 27.8308) (-32.4105, 27.675) (-31.9184, 26.9916) (-31.7626, 26.753) knots 0 0 0 0 1 1 1 1
  line L656 (-31.7626, 26.753) -> (-31.5918, 26.7541)
  spline S1227 degree 3 poles (-31.5918, 26.7541) (-31.7111, 26.9099) (-32.0902, 27.4794) (-32.1364, 27.5568) knots 0 0 0 0 1 1 1 1
  spline S1228 degree 3 poles (-32.1364, 27.5568) (-32.187, 27.6406) (-32.0752, 27.9147) (-32.0419, 27.6793) knots 0 0 0 0 1 1 1 1
  spline S1229 degree 3 poles (-32.0419, 27.6793) (-32.0087, 27.4472) (-31.5273, 26.9142) (-31.4295, 26.7552) knots 0 0 0 0 1 1 1 1
  line L657 (-31.4295, 26.7552) -> (-31.2481, 26.7584)
  spline S1230 degree 3 poles (-31.2481, 26.7584) (-31.3276, 26.9067) (-31.6111, 27.286) (-31.6616, 27.444) knots 0 0 0 0 1 1 1 1
  spline S1231 degree 3 poles (-31.6616, 27.444) (-31.7175, 27.6181) (-31.6391, 27.5955) (-31.5832, 27.4945) knots 0 0 0 0 1 1 1 1
  spline S1232 degree 3 poles (-31.5832, 27.4945) (-31.4105, 27.2428) (-31.2267, 26.999) (-31.0321, 26.7638) knots 0 0 0 0 1 1 1 1
  line L658 (-31.0321, 26.7638) -> (-30.9021, 26.7681)
  spline S1233 degree 3 poles (-30.9021, 26.7681) (-30.9837, 26.8949) (-31.1588, 27.1592) (-31.2019, 27.2377) knots 0 0 0 0 1 1 1 1
  spline S1234 degree 3 poles (-31.2019, 27.2377) (-31.2534, 27.3269) (-31.2147, 27.3945) (-31.1567, 27.3097) knots 0 0 0 0 1 1 1 1
  spline S1235 degree 3 poles (-31.1567, 27.3097) (-31.1019, 27.2258) (-30.7378, 26.8906) (-30.6592, 26.7842) knots 0 0 0 0 1 1 1 1
  line L659 (-30.6592, 26.7842) -> (-30.655, 26.7788)
  line L660 (-30.655, 26.7788) -> (-30.4928, 26.7896)
  spline S1236 degree 3 poles (-30.4928, 26.7896) (-30.5498, 26.8723) (-30.6357, 26.9722) (-30.7334, 27.07) knots 0 0 0 0 1 1 1 1
  spline S1237 degree 3 poles (-30.7334, 27.07) (-30.8558, 27.1925) (-30.7442, 27.2935) (-30.683, 27.1979) knots 0 0 0 0 1 1 1 1
  spline S1238 degree 3 poles (-30.683, 27.1979) (-30.6293, 27.113) (-30.3682, 26.9239) (-30.2522, 26.81) knots 0 0 0 0 1 1 1 1
  line L661 (-30.2522, 26.81) -> (-30.193, 26.8164)
  line L662 (-30.193, 26.8164) -> (-30.1135, 26.8261)
  spline S1239 degree 3 poles (-30.1135, 26.8261) (-30.1791, 26.9303) (-30.2683, 27.0625) (-30.3145, 27.1313) knots 0 0 0 0 1 1 1 1
  spline S1240 degree 3 poles (-30.3145, 27.1313) (-30.3757, 27.2205) (-30.3865, 27.3215) (-30.3252, 27.2538) knots 0 0 0 0 1 1 1 1
  spline S1241 degree 3 poles (-30.3252, 27.2538) (-30.185, 27.1158) (-30.0392, 26.9839) (-29.8879, 26.8583) knots 0 0 0 0 1 1 1 1
  line L663 (-29.8879, 26.8583) -> (-29.7483, 26.8798)
  spline S1242 degree 3 poles (-29.7483, 26.8798) (-29.8654, 27.0475) (-30.0415, 27.2871) (-30.1018, 27.3548) knots 0 0 0 0 1 1 1 1
  spline S1243 degree 3 poles (-30.1018, 27.3548) (-30.191, 27.4558) (-30.1135, 27.5224) (-30.0459, 27.4386) knots 0 0 0 0 1 1 1 1
  spline S1244 degree 3 poles (-30.0459, 27.4386) (-29.9933, 27.3752) (-29.7181, 27.0904) (-29.5442, 26.911) knots 0 0 0 0 1 1 1 1
  line L664 (-29.5442, 26.911) -> (-29.3421, 26.9411)
  spline S1245 degree 3 poles (-29.3421, 26.9411) (-29.3819, 26.997) (-29.4271, 27.0539) (-29.4744, 27.1087) knots 0 0 0 0 1 1 1 1
  spline S1246 degree 3 poles (-29.4744, 27.1087) (-29.5528, 27.1979) (-29.4689, 27.243) (-29.3905, 27.1646) knots 0 0 0 0 1 1 1 1
  spline S1247 degree 3 poles (-29.3905, 27.1646) (-29.3184, 27.096) (-29.2434, 27.0304) (-29.166, 26.9679) knots 0 0 0 0 1 1 1 1
  line L665 (-29.166, 26.9679) -> (-28.9641, 26.9959)
  spline S1248 degree 3 poles (-28.9641, 26.9959) (-29.0522, 27.1109) (-29.2444, 27.2828) (-29.3346, 27.3827) knots 0 0 0 0 1 1 1 1
  spline S1249 degree 3 poles (-29.3346, 27.3827) (-29.441, 27.4999) (-29.4013, 27.5568) (-29.3229, 27.4773) knots 0 0 0 0 1 1 1 1
  spline S1250 degree 3 poles (-29.3229, 27.4773) (-29.2595, 27.415) (-28.9824, 27.1549) (-28.8318, 27.0131) knots 0 0 0 0 1 1 1 1
  line L666 (-28.8318, 27.0131) -> (-28.6826, 27.0324)
  spline S1251 degree 3 poles (-28.6826, 27.0324) (-28.7599, 27.1506) (-28.9404, 27.4236) (-29.0092, 27.5128) knots 0 0 0 0 1 1 1 1
  spline S1252 degree 3 poles (-29.0092, 27.5128) (-29.0876, 27.6127) (-29.037, 27.6922) (-28.9533, 27.5794) knots 0 0 0 0 1 1 1 1
  spline S1253 degree 3 poles (-28.9533, 27.5794) (-28.8856, 27.488) (-28.5718, 27.2076) (-28.4076, 27.0614) knots 0 0 0 0 1 1 1 1
  line L667 (-28.4076, 27.0614) -> (-28.2335, 27.0754)
  spline S1254 degree 3 poles (-28.2335, 27.0754) (-28.3484, 27.2248) (-28.6363, 27.6245) (-28.7019, 27.7137) knots 0 0 0 0 1 1 1 1
  spline S1255 degree 3 poles (-28.7019, 27.7137) (-28.7739, 27.8147) (-28.7341, 27.8427) (-28.6687, 27.776) knots 0 0 0 0 1 1 1 1
  spline S1256 degree 3 poles (-28.6687, 27.776) (-28.456, 27.5496) (-28.2469, 27.3199) (-28.0413, 27.0872) knots 0 0 0 0 1 1 1 1
  line L668 (-28.0413, 27.0872) -> (-27.865, 27.0937)
  spline S1257 degree 3 poles (-27.865, 27.0937) (-27.981, 27.2624) (-28.3281, 27.6976) (-28.4107, 27.776) knots 0 0 0 0 1 1 1 1
  spline S1258 degree 3 poles (-28.4107, 27.776) (-28.5064, 27.8652) (-28.4173, 27.9104) (-28.3378, 27.8427) knots 0 0 0 0 1 1 1 1
  spline S1259 degree 3 poles (-28.3378, 27.8427) (-28.27, 27.7836) (-27.8392, 27.2667) (-27.6802, 27.0947) knots 0 0 0 0 1 1 1 1
  spline S1260 degree 3 poles (-27.6802, 27.0947) (-27.6243, 27.0947) (-27.5675, 27.0937) (-27.5116, 27.0915) knots 0 0 0 0 1 1 1 1
  spline S1261 degree 3 poles (-27.5116, 27.0915) (-27.6136, 27.2678) (-27.9177, 27.6417) (-28.0197, 27.7868) knots 0 0 0 0 1 1 1 1
  spline S1262 degree 3 poles (-28.0197, 27.7868) (-28.1432, 27.9609) (-28.0595, 27.949) (-27.9649, 27.8534) knots 0 0 0 0 1 1 1 1
  spline S1263 degree 3 poles (-27.9649, 27.8534) (-27.8812, 27.7696) (-27.4944, 27.2989) (-27.3172, 27.0797) knots 0 0 0 0 1 1 1 1
  spline S1264 degree 3 poles (-27.3172, 27.0797) (-27.2432, 27.0745) (-27.1693, 27.067) (-27.0958, 27.0571) knots 0 0 0 0 1 1 1 1
  line L669 (-27.0958, 27.0571) -> (-27.1001, 27.0668)
  spline S1265 degree 3 poles (-27.1001, 27.0668) (-27.2076, 27.2398) (-27.4697, 27.6987) (-27.6104, 27.833) knots 0 0 0 0 1 1 1 1
  spline S1266 degree 3 poles (-27.6104, 27.833) (-27.7489, 27.9673) (-27.6492, 28.0178) (-27.5534, 27.8996) knots 0 0 0 0 1 1 1 1
  spline S1267 degree 3 poles (-27.5534, 27.8996) (-27.4718, 27.7986) (-27.0496, 27.2559) (-26.8573, 27.0141) knots 0 0 0 0 1 1 1 1